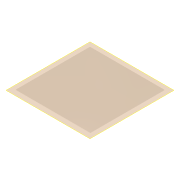
# Autodesk Inventor part: 00_coverglass_18mm
Saved by Autodesk Inventor 2022 (Build 260153000, 153)
## iProperties
Created: 2021-12-21
Part Number: 00_coverglass_18mm
Material: Generisch
Document SubType Name: Modeling
Designer: diederichbenedict
Density: 1 g/cm^3
Appearance: Polycarbonat - klar
Author: diederichbenedict
Autodesk Inventor part; units mm, degrees
ref_plane "YZ Plane" through (0, 0, 0) normal (1, 0, 0) x (0, 1, 0)
ref_plane "XZ Plane" through (0, 0, 0) normal (0, 1, 0) x (-1, 0, 0)
ref_plane "XY Plane" through (0, 0, 0) normal (0, 0, 1) x (1, 0, 0)
ref_plane "Arbeitsebene1" through (19.9549, -12.8968, -0.043) normal (0, 1, 0) x (-1, 0, 0)
sketch "Skizze1" plane through (19.9549, -12.8968, -0.043) normal (0, 1, 0) x (-1, 0, 0)
  line L0 (9.25, 9.25) -> (-9.25, 9.25) projected
  line L1 (-9.25, 9.25) -> (-9.25, -9.25) projected
  line L2 (-9.25, -9.25) -> (9.25, -9.25) projected
  line L3 (9.25, -9.25) -> (9.25, 9.25) projected
  line L4 (8.5, 8.5) -> (8.5, -8.5) projected
  line L5 (8.5, -8.5) -> (-8.5, -8.5) projected
  line L6 (-8.5, -8.5) -> (-8.5, 8.5) projected
  line L7 (-8.5, 8.5) -> (8.5, 8.5) projected
  line L8 (-9, -9) -> (9, -9)
  line L9 (9, -9) -> (9, 9)
  line L10 (9, 9) -> (-9, 9)
  line L11 (-9, 9) -> (-9, -9)
  line L12 (-9, -9) -> (9, 9) construction
  line L13 (9, -9) -> (-9, 9) construction
  point P0 (19.9549, 0.043)
  point P1 (0, 0)
  dimension "d0" = 18
  dimension "d1" = 18
  constraints: 12 end point, 2 midpoint, 2 parallel, 1 horizontal, 1 perpendicular
  measures "d0" distance of L10.end L9.end
  measures "d1" distance of L9.end L8.end
extrude "Extrusion1" add sketch "Skizze1" along normal blind 0.125 contours L4 L5 L6 L7 | L11 L10 L9 L8
